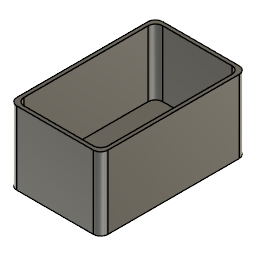
bin (~recovered) (Autodesk Fusion 360 design; units mm, degrees)
Autodesk Fusion 360 part; units mm, degrees
sketch "Sketch1" plane through (0, 0, 0) normal (0, 0, 1) x (1, 0, 0)
  line L0 (-125, 200) -> (125, 200)
  line L1 (125, 200) -> (125, -200)
  line L2 (125, -200) -> (-125, -200)
  line L3 (-125, -200) -> (-125, 200)
  dimension "d1" = 250
  dimension "d2" = 400
  constraint horizontal L0
  constraint perpendicular L0 L1
  constraint parallel L0 L2
  constraint parallel L1 L3
  measures "d1" distance of L1.end L2.end
  measures "d2" distance of L0.end L1.end
extrude "Extrude1" add sketch "Sketch1" along normal blind 200
sketch "Sketch2" plane through (0, 0, 200) normal (0, 0, 1) x (-1, 0, 0)
  line L0 (125, 200) -> (-125, 200)
  line L1 (-125, 200) -> (-125, -200)
  line L2 (-125, -200) -> (125, -200)
  line L3 (125, -200) -> (125, 200)
  line L4 (115, -190) -> (-115, -190)
  line L5 (-115, -190) -> (-115, 190)
  line L6 (-115, 190) -> (115, 190)
  line L7 (115, 190) -> (115, -190)
  dimension "d5" = 230
  dimension "d6" = 380
  constraint horizontal L4
  constraint perpendicular L4 L5
  constraint parallel L4 L6
  constraint parallel L5 L7
  measures "d5" distance of L5.end L6.end
  measures "d6" distance of L4.end L5.end
extrude "Extrude2" cut sketch "Sketch2" against normal blind 180 contours L4 L5 L6 L7
fillet "Fillet1" radius 20 4 edges at (-125, -200, 100) (125, -200, 100) (125, 200, 100) (-125, 200, 100)
fillet "Fillet2" radius 20 4 edges at (115, -190, 110) (-115, -190, 110) (115, 190, 110) (-115, 190, 110)
